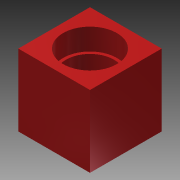
# Autodesk Inventor part: pinch_wheel_hobbing_jig
Saved by Autodesk Inventor 2014 (Build 180170000, 170)
## iProperties
Created: 2014-01-05
Part Number: pinch_wheel_hobbing_jig
Material: Generic
Document SubType Name: Modeling
Designer: caleb
Density: 1 g/cm^3
Appearance: Light Red
Author: caleb
Autodesk Inventor part; units mm, degrees
ref_plane "YZ Plane" through (0, 0, 0) normal (1, 0, 0) x (0, 1, 0)
sketch "Sketch1" plane through (0, 0, 0) normal (0, 0, 1) x (1, 0, 0)
  circle A0 centre (0, 0) radius 11.25
  line L0 (-15, -15) -> (15, -15)
  line L1 (15, -15) -> (15, 15)
  line L2 (15, 15) -> (-15, 15)
  line L3 (-15, 15) -> (-15, -15)
  point P0 (-15, 0)
  point P1 (0, 15)
  dimension "d0" = 22.5
  dimension "d1" = 30
  constraints: 8 end point, 2 midpoint, 2 parallel, 2 perpendicular, 1 centre point, 1 coincident, 1 horizontal, 1 horizontal alignment, 1 vertical alignment
  measures "d0" diameter of A0
  measures "d1" distance of L2.end L0.start
extrude "Extrusion1" add sketch "Sketch1" along normal blind 30
ref_plane "Work Plane1" through (0, 0, 21) normal (0, 0, 1) x (1, 0, 0)
ref_plane "Work Plane2" through (0, 0, 9) normal (0, 0, -1) x (-1, 0, 0)
sketch "Sketch2" plane through (0, 0, 21) normal (0, 0, 1) x (1, 0, 0)
  circle A0 centre (0, 0) radius 10
  circle A1 centre (0, 0) radius 11.25 projected
  dimension "d6" = 20
  constraints: 1 centre point, 1 coincident
  measures "d6" diameter of A0
extrude "Extrusion2" add sketch "Sketch2" against normal up to surface (12 mm away)
sketch "Sketch3" plane through (0, 0, 0) normal (1, 0, 0) x (0, 1, 0)
  line L0 (15, 30) -> (15, 0) projected
  line L1 (15, 0) -> (11.25, 0) projected
  line L2 (11.25, 0) -> (11.25, 9) projected
  line L3 (11.25, 9) -> (10, 9) projected
  line L4 (10, 9) -> (10, 21) projected
  line L5 (10, 21) -> (11.25, 21) projected
  line L6 (11.25, 21) -> (11.25, 30) projected
  line L7 (11.25, 30) -> (15, 30) projected
  line L8 (-15, 0) -> (-15, 30) projected
  line L9 (-15, 30) -> (-11.25, 30) projected
  line L10 (-11.25, 30) -> (-11.25, 21) projected
  line L11 (-11.25, 21) -> (-10, 21) projected
  line L12 (-10, 21) -> (-10, 9) projected
  line L13 (-10, 9) -> (-11.25, 9) projected
  line L14 (-11.25, 9) -> (-11.25, 0) projected
  line L15 (-11.25, 0) -> (-15, 0) projected
  line L16 (-10, 9) -> (-11.25, 7.75)
  line L17 (0, -4) -> (0, 24) projected
  point P0 (0, 0)
  dimension "d9" = 45
  constraints: 2 end point, 1 point on line
  measures "d9" angle of L14 L16
revolve "Revolution1" add sketch "Sketch3" angle 360 about axis through (0, 0, -10) along (0, 0, 1) contours L14 L13 L16
equation "\"d0\" = od + hole_oversize"
equation "\"d6\" = damax"
equation "\"id\" = 8"
equation "\"od\" = 22"
equation "\"hole_oversize\" = 0.5"
equation "\"post_oversize\" = 0"
equation "\"bearing_width\" = 9"
equation "\"d4\" = -bearing_width"
equation "\"d5\" = -bearing_width"
equation "\"damax\" = 20"
body "Solid1"
